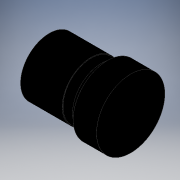
# Autodesk Inventor part: 00_Eyepiece_WF20x 23,2mm
Saved by Autodesk Inventor 2019 (Build 230136000, 136)
## iProperties
Created: 2017-06-09
Part Number: 00_Eyepiece_WF20x 23,2mm
Material: Generisch
Document SubType Name: Modeling
Designer: diederichbenedict
Density: 1 g/cm^3
Appearance: Schwarz
Author: diederichbenedict
Autodesk Inventor part; units mm, degrees
ref_plane "YZ Plane" through (0, 0, 0) normal (1, 0, 0) x (0, 1, 0)
ref_plane "XZ Plane" through (0, 0, 0) normal (0, 1, 0) x (-1, 0, 0)
ref_plane "XY Plane" through (0, 0, 0) normal (0, 0, 1) x (1, 0, 0)
sketch "Skizze1" plane through (0, 0, 0) normal (0, 0, 1) x (1, 0, 0)
  line L0 (0, 0) -> (16.6, 0)
  line L1 (16.6, 0) -> (16.6, 11.45)
  line L2 (16.6, 11.45) -> (0, 11.45)
  line L3 (0, 11.45) -> (0, 0)
  line L4 (16.6, 0) -> (20.7, 0)
  line L5 (20.7, 0) -> (20.7, 11.15)
  line L6 (20.7, 11.15) -> (16.6, 11.15)
  line L7 (16.6, 11.15) -> (16.6, 0)
  line L8 (20.7, 0) -> (23.1, 0)
  line L9 (23.1, 0) -> (23.1, 11.45)
  line L10 (23.1, 11.45) -> (20.7, 11.45)
  line L11 (20.7, 11.45) -> (20.7, 0)
  line L12 (23.1, 0) -> (32.4, 0)
  line L13 (32.4, 0) -> (32.4, 13.6)
  line L14 (32.4, 13.6) -> (23.1, 13.6)
  line L15 (23.1, 13.6) -> (23.1, 0)
  dimension "d1" = 11.45
  dimension "d2" = 4.1
  dimension "d3" = 11.15
  dimension "d4" = 2.4
  dimension "d5" = 9.3
  dimension "d6" = 13.6
  dimension "d8" = 32.4
  constraints: 32 end point, 8 parallel, 4 horizontal, 4 perpendicular, 1 point on line
  measures "d1" distance of L1.end L0.end
  measures "d2" distance of L6.end L5.end
  measures "d3" distance of L5.end L4.end
  measures "d4" distance of L10.end L9.end
  measures "d5" distance of L14.end L13.end
  measures "d6" distance of L13.end L12.end
  measures "d8" distance between parallel lines of L3 L13
revolve "Umdrehung1" add sketch "Skizze1" angle 360 about axis through (0, 0, 0) along (1, 0, 0)
